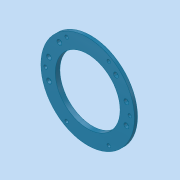
# Autodesk Inventor part: forwardBallastSealingWallRear
Saved by Autodesk Inventor 2017 (Build 210142000, 142)
## iProperties
Created: 2016-11-26
Part Number: forwardBallastSealingWallRear
Material: ABS Plastic
Document SubType Name: Modeling
Designer: techn
Density: 1.06 g/cm^3
Appearance: Sky Blue Dark
Mass: 12.5682 g
Surface Area: 98.4279 cm^2
Volume: 11.8568 cm^3
Author: techn
Autodesk Inventor part; units mm, degrees
ref_plane "YZ Plane" through (0, 0, 0) normal (1, 0, 0) x (0, 1, 0)
ref_plane "XZ Plane" through (0, 0, 0) normal (0, 1, 0) x (-1, 0, 0)
ref_plane "XY Plane" through (0, 0, 0) normal (0, 0, 1) x (1, 0, 0)
sketch "Sketch1" plane through (0, 0, 0) normal (0, 0, 1) x (1, 0, 0)
  circle A0 centre (0, 0) radius 47.625
  line L0 (0, 0) -> (21.4313, 37.12)
  line L1 (0, 0) -> (42.8625, 0) construction
  circle A1 centre (21.4313, 37.12) radius 1.8415
  circle A2 centre (-21.4312, 37.12) radius 1.8415
  circle A3 centre (-42.8625, 0) radius 1.8415
  circle A4 centre (-21.4313, -37.12) radius 1.8415
  circle A5 centre (21.4312, -37.12) radius 1.8415
  circle A6 centre (42.8625, 0) radius 1.8415
  dimension "d0" = 95.25
  dimension "d1" = 42.8625
  dimension "d2" = 60
  dimension "d3" = 3.683
  dimension "d6" = 360
  constraints: 7 centre point, 4 end point, 2 coincident, 1 equal length, 1 horizontal, 13 other
  measures "d0" diameter of A0
  measures "d1" distance of L0.start L0.end
  measures "d2" angle of L1 L0
  measures "d3" diameter of A1
extrude "Extrusion1" add sketch "Sketch1" along normal blind 3.175
sketch "Sketch3" plane through (0, 0, 0) normal (0, 0, -1) x (-1, 0, 0)
  circle A0 centre (0, 0) radius 41.275
  circle A1 centre (0, 0) radius 34.6075
  dimension "d10" = 82.55
  dimension "d11" = 69.215
  constraints: 2 centre point, 2 coincident
  measures "d10" diameter of A0
  measures "d11" diameter of A1
extrude "Extrusion2" add sketch "Sketch3" along normal blind 1.5875 contours A1
sketch "Sketch6" plane through (0, 0, -1.5875) normal (0, 0, -1) x (-1, 0, 0)
  circle A0 centre (0, 0) radius 33.02
  dimension "d27" = 66.04
  constraints: 1 centre point, 1 coincident
  measures "d27" diameter of A0
extrude "Extrusion4" cut sketch "Sketch6" against normal blind 25.4
sketch "Sketch8" plane through (0, 0, 3.175) normal (0, 0, 1) x (1, 0, 0)
  line L0 (0, 0) -> (39.3779, 10.5513)
  line L1 (0, 0) -> (40.767, 0) construction
  circle A0 centre (39.3779, 10.5513) radius 2.54
  line L2 (0, 0) -> (0, 8.7749)
  circle A1 centre (39.3779, -10.5513) radius 2.54
  circle A2 centre (-39.3779, 10.5513) radius 2.54
  circle A3 centre (-39.3779, -10.5513) radius 2.54
  circle A4 centre (21.4313, 37.12) radius 1.8415 projected
  line L3 (21.4313, 37.12) -> (0, 0)
  circle A5 centre (28.8266, 28.8266) radius 2.54
  line L4 (28.8266, 28.8266) -> (0, 0)
  circle A6 centre (-28.8266, 28.8266) radius 2.54
  dimension "d30" = 40.767
  dimension "d31" = 15
  dimension "d32" = 5.08
  dimension "d35" = 15
  dimension "d36" = 40.767
  dimension "d37" = 5.08
  constraints: 10 end point, 6 centre point, 4 symmetric about line, 1 coincident, 1 equal length, 1 horizontal, 1 vertical, 4 other
  measures "d30" distance of L0.start L0.end
  measures "d31" angle of L1 L0
  measures "d32" diameter of A0
  measures "d35" angle of L4 L3
  measures "d36" distance of L4.start L0.start
  measures "d37" diameter of A5
extrude "Extrusion5" cut sketch "Sketch8" against normal blind 25.4 contours A0 | A1 | A2 | A3
extrude "Extrusion6" cut sketch "Sketch8" against normal blind 25.4 contours A5 | A6
sketch "Sketch9" plane through (0, 0, 3.175) normal (0, 0, 1) x (1, 0, 0)
  circle A0 centre (0, 0) radius 47.625
  circle A1 centre (0, 0) radius 47.117
  dimension "d40" = 95.25
  dimension "d41" = 94.234
  constraints: 2 centre point, 2 coincident
  measures "d40" diameter of A0
  measures "d41" diameter of A1
extrude "PRINT_FEATURE_1" [suppressed]
equation "\"d35\" = d31"
equation "\"d36\" = d30"
equation "\"d37\" = d32"
body "Solid1"
